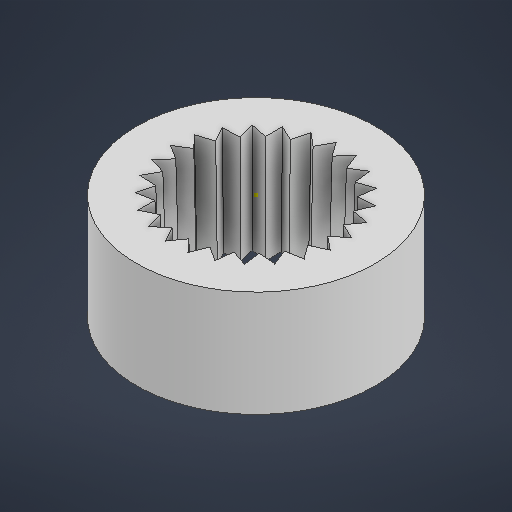
# Autodesk Inventor part: OMG_servo_head(1deg)
Saved by Autodesk Inventor 2026.1 (Build 301233020, 233B)
## iProperties
Created: 2026-02-22
Part Number: OMG_servo_head(1deg)
Material: Generic
Document SubType Name: Modeling
Designer: Lars
Density: 1 g/cm^3
Appearance: Default
Author: Lars
Autodesk Inventor part; units mm, degrees
ref_plane "YZ Plane" through (0, 0, 0) normal (1, 0, 0) x (0, 1, 0)
ref_plane "XZ Plane" through (0, 0, 0) normal (0, 1, 0) x (-1, 0, 0)
ref_plane "XY Plane" through (0, 0, 0) normal (0, 0, 1) x (1, 0, 0)
sketch "Sketch1" plane through (0, 0, 0) normal (0, 1, 0) x (-1, 0, 0)
  circle A0 centre (0, 0) radius 3.1 construction
  circle A1 centre (0, 0) radius 2.6 construction
  line L0 (3.1, 0) -> (2.5795, 0.3259)
  line L1 (3.1, 0) -> (2.5795, -0.3259)
  line L2 (3.1, 0) -> (2.6, 0) construction
  line L3 (3.0026, 0.7709) -> (2.4174, 0.9571)
  line L4 (3.0026, 0.7709) -> (2.5795, 0.3259)
  line L5 (2.7166, 1.4934) -> (2.1034, 1.5282)
  line L6 (2.7166, 1.4934) -> (2.4174, 0.9571)
  line L7 (2.2598, 2.1221) -> (1.6573, 2.0033)
  line L8 (2.2598, 2.1221) -> (2.1034, 1.5282)
  line L9 (1.6611, 2.6174) -> (1.107, 2.3526)
  line L10 (1.6611, 2.6174) -> (1.6573, 2.0033)
  line L11 (0.958, 2.9483) -> (0.4872, 2.5539)
  line L12 (0.958, 2.9483) -> (1.107, 2.3526)
  line L13 (0.1947, 3.0939) -> (-0.1633, 2.5949)
  line L14 (0.1947, 3.0939) -> (0.4872, 2.5539)
  line L15 (-0.5809, 3.0451) -> (-0.8034, 2.4727)
  line L16 (-0.5809, 3.0451) -> (-0.1633, 2.5949)
  line L17 (-1.3199, 2.805) -> (-1.3931, 2.1953)
  line L18 (-1.3199, 2.805) -> (-0.8034, 2.4727)
  line L19 (-1.976, 2.3886) -> (-1.8953, 1.7798)
  line L20 (-1.976, 2.3886) -> (-1.3931, 2.1953)
  line L21 (-2.508, 1.8221) -> (-2.2784, 1.2526)
  line L22 (-2.508, 1.8221) -> (-1.8953, 1.7798)
  line L23 (-2.8823, 1.1412) -> (-2.5183, 0.6466)
  line L24 (-2.8823, 1.1412) -> (-2.2784, 1.2526)
  line L25 (-3.0756, 0.3885) -> (-2.6, 0)
  line L26 (-3.0756, 0.3885) -> (-2.5183, 0.6466)
  line L27 (-3.0756, -0.3885) -> (-2.5183, -0.6466)
  line L28 (-3.0756, -0.3885) -> (-2.6, 0)
  line L29 (-2.8823, -1.1412) -> (-2.2784, -1.2526)
  line L30 (-2.8823, -1.1412) -> (-2.5183, -0.6466)
  line L31 (-2.508, -1.8221) -> (-1.8953, -1.7798)
  line L32 (-2.508, -1.8221) -> (-2.2784, -1.2526)
  line L33 (-1.976, -2.3886) -> (-1.3931, -2.1953)
  line L34 (-1.976, -2.3886) -> (-1.8953, -1.7798)
  line L35 (-1.3199, -2.805) -> (-0.8034, -2.4727)
  line L36 (-1.3199, -2.805) -> (-1.3931, -2.1953)
  line L37 (-0.5809, -3.0451) -> (-0.1633, -2.5949)
  line L38 (-0.5809, -3.0451) -> (-0.8034, -2.4727)
  line L39 (0.1947, -3.0939) -> (0.4872, -2.5539)
  line L40 (0.1947, -3.0939) -> (-0.1633, -2.5949)
  line L41 (0.958, -2.9483) -> (1.107, -2.3526)
  line L42 (0.958, -2.9483) -> (0.4872, -2.5539)
  line L43 (1.6611, -2.6174) -> (1.6573, -2.0033)
  line L44 (1.6611, -2.6174) -> (1.107, -2.3526)
  line L45 (2.2598, -2.1221) -> (2.1034, -1.5282)
  line L46 (2.2598, -2.1221) -> (1.6573, -2.0033)
  line L47 (2.7166, -1.4934) -> (2.4174, -0.9571)
  line L48 (2.7166, -1.4934) -> (2.1034, -1.5282)
  line L49 (3.0026, -0.7709) -> (2.5795, -0.3259)
  line L50 (3.0026, -0.7709) -> (2.4174, -0.9571)
  circle A2 centre (0, 0) radius 4.5
  point P0 (2.4174, 0.9571)
  point P1 (-0.1633, 2.5949)
  point P2 (-0.8034, 2.4727)
  point P3 (-2.6, 0)
  point P4 (-2.5183, -0.6466)
  point P5 (-0.1633, -2.5949)
  dimension "d0" = 6.2
  dimension "d1" = 0.5
  dimension "d3" = 0.5
  dimension "d6" = 360
  dimension "d11" = 9
  constraints: 102 end point, 3 coincident, 3 point on circle, 2 centre point, 1 horizontal, 1 horizontal alignment, 129 other
  measures "d3" distance of L0.start L2.end
  measures "d11" diameter of A2
extrude "Extrusion1" add sketch "Sketch1" along normal blind 4 contours L1 L49 L50 L47 L48 L45 L46 L43 L44 L41 L42 L39 L40 L37 L38 L35 L36 L33 L34 L31 L32 L29 L30 L27 L28 L25 L26 L23 L24 L21 L22 L19 L20 L17 L18 L15 L16 L13 L14 L11 L12 L9 L10 L7 L8 L5 L6 L3 L4 L0 | A2
extrude "Extrusion2" cut sketch "Sketch1" along normal blind 4 draft 1 contours L1 L49 L50 L47 L48 L45 L46 L43 L44 L41 L42 L39 L40 L37 L38 L35 L36 L33 L34 L31 L32 L29 L30 L27 L28 L25 L26 L23 L24 L21 L22 L19 L20 L17 L18 L15 L16 L13 L14 L11 L12 L9 L10 L7 L8 L5 L6 L3 L4 L0
sketch "Sketch3" plane through (0, 4, 0) normal (0, 1, 0) x (1, 0, 0)
  point P0 (0, 0)
equation "\"d3\" = d1"
body "Solid1"
